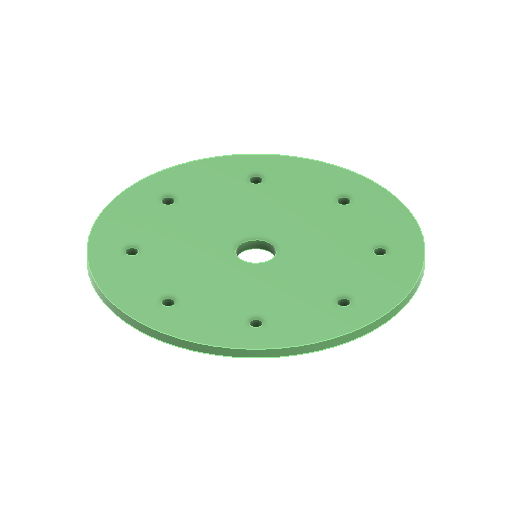
# Autodesk Inventor part: CUT_FR4_Bottom_Cone_PCB
Saved by Autodesk Inventor 2026.1 (Build 301233000, 233)
## iProperties
Created: 2025-06-19
Part Number: CUT_FR4_Bottom_Cone_PCB
Material: Generic
Document SubType Name: Modeling
Designer: User
Density: 1 g/cm^3
Appearance: Smooth - Dark Forest Green
Author: User
Autodesk Inventor part; units mm, degrees
ref_plane "YZ Plane" through (0, 0, 0) normal (1, 0, 0) x (0, 1, 0)
ref_plane "XZ Plane" through (0, 0, 0) normal (0, 1, 0) x (-1, 0, 0)
ref_plane "XY Plane" through (0, 0, 0) normal (0, 0, 1) x (1, 0, 0)
sketch "Sketch1" plane through (0, 0, 0) normal (0, 1, 0) x (-1, 0, 0)
  circle A0 centre (0, 0) radius 25
  circle A1 centre (0, 0) radius 3
  circle A2 centre (0, 18.36) radius 1
  circle A3 centre (-12.9825, 12.9825) radius 1
  circle A4 centre (-18.36, 0) radius 1
  circle A5 centre (-12.9825, -12.9825) radius 1
  circle A6 centre (0, -18.36) radius 1
  circle A7 centre (12.9825, -12.9825) radius 1
  circle A8 centre (18.36, 0) radius 1
  circle A9 centre (12.9825, 12.9825) radius 1
  dimension "d0" = 50
  dimension "d1" = 6
  dimension "d2" = 2
  dimension "d3" = 18.36
  dimension "d6" = 360
  constraints: 10 centre point, 2 coincident, 17 other
  measures "d0" diameter of A0
  measures "d1" diameter of A1
  measures "d2" diameter of A2
  measures "d3" distance of point (0, 0) A2.centre
extrude "Extrusion1" add sketch "Sketch1" along normal blind 1.6
body "Solid1"
